Autodesk Fusion 360 part; units mm, degrees
(part 2 of 2)
  line L893 (352.3496, 85.2824) -> (352.3435, 85.227)
  line L894 (352.3793, 85.4468) -> (352.3675, 85.3923)
  line L895 (352.3576, 85.3375) -> (352.3496, 85.2824)
  line L896 (352.7563, 83.9952) -> (352.7945, 83.9547)
  line L897 (352.4662, 85.7111) -> (352.4452, 85.6595)
  line L898 (353.1622, 86.4835) -> (353.114, 86.4555)
  line L899 (352.618, 84.1698) -> (352.6503, 84.1244)
  line L900 (352.3393, 85.1714) -> (352.337, 85.1158)
  line L901 (352.7945, 83.9547) -> (352.8342, 83.9156)
  line L902 (352.5309, 84.3124) -> (352.5583, 84.2639)
  line L903 (352.3367, 85.06) -> (352.3383, 85.0043)
  line L904 (352.6286, 86.0027) -> (352.5974, 85.9565)
  line L905 (353.0206, 86.3947) -> (352.9756, 86.3619)
  line L906 (352.4386, 84.5151) -> (352.459, 84.4632)
  line L907 (354.279, 83.5057) -> (354.3337, 83.5183)
  line L908 (273.0588, 85.3008) -> (273.0502, 85.3558)
  line L909 (355.0618, 83.9218) -> (355.1015, 83.9615)
  line L910 (354.8899, 83.7776) -> (354.9347, 83.8114)
  line L911 (354.6496, 83.6333) -> (354.6996, 83.6587)
  line L912 (355.544, 84.9105) -> (355.5489, 84.9664)
  line L913 (353.7225, 83.4859) -> (353.7778, 83.4792)
  line L914 (354.3879, 83.5328) -> (354.4416, 83.5492)
  line L915 (354.7487, 83.686) -> (354.7969, 83.7149)
  line L916 (355.2119, 84.0886) -> (355.2457, 84.1334)
  line L917 (355.5518, 85.0225) -> (355.5528, 85.0786)
  line L918 (353.3986, 83.5661) -> (353.4513, 83.5481)
  line L919 (355.505, 84.6896) -> (355.5176, 84.7443)
  line L920 (273.0656, 85.2455) -> (273.0588, 85.3008)
  line L921 (355.5371, 84.8548) -> (355.544, 84.9105)
  line L922 (353.5046, 83.5319) -> (353.5585, 83.5176)
  line L923 (273.0704, 85.19) -> (273.0656, 85.2455)
  line L924 (355.5176, 84.7443) -> (355.5284, 84.7994)
  line L925 (353.9447, 83.4705) -> (354.0008, 83.4715)
  line L926 (355.1397, 84.0026) -> (355.1766, 84.045)
  line L927 (353.4513, 83.5481) -> (353.5046, 83.5319)
  line L928 (354.1685, 83.4862) -> (354.2239, 83.4949)
  line L929 (355.39, 84.3737) -> (355.4138, 84.4245)
  line L930 (355.2457, 84.1334) -> (355.2779, 84.1794)
  line L931 (355.5284, 84.7994) -> (355.5371, 84.8548)
  line L932 (354.3337, 83.5183) -> (354.3879, 83.5328)
  line L933 (355.5489, 84.9664) -> (355.5518, 85.0225)
  line L934 (355.2779, 84.1794) -> (355.3084, 84.2265)
  line L935 (355.4138, 84.4245) -> (355.4357, 84.4762)
  line L936 (354.9784, 83.8467) -> (355.0207, 83.8836)
  line L937 (354.1128, 83.4793) -> (354.1685, 83.4862)
  line L938 (354.2239, 83.4949) -> (354.279, 83.5057)
  line L939 (354.6996, 83.6587) -> (354.7487, 83.686)
  line L940 (353.7778, 83.4792) -> (353.8333, 83.4744)
  line L941 (355.4357, 84.4762) -> (355.4558, 84.5286)
  line L942 (353.5585, 83.5176) -> (353.6128, 83.5051)
  line L943 (354.4416, 83.5492) -> (354.4947, 83.5675)
  line L944 (354.9347, 83.8114) -> (354.9784, 83.8467)
  line L945 (354.4947, 83.5675) -> (354.5471, 83.5876)
  line L946 (353.3465, 83.5859) -> (353.3986, 83.5661)
  line L947 (354.5988, 83.6095) -> (354.6496, 83.6333)
  line L948 (355.3084, 84.2265) -> (355.3373, 84.2746)
  line L949 (353.6675, 83.4946) -> (353.7225, 83.4859)
  line L950 (355.4558, 84.5286) -> (355.4741, 84.5817)
  line L951 (354.0008, 83.4715) -> (354.0569, 83.4744)
  line L952 (354.0569, 83.4744) -> (354.1128, 83.4793)
  line L953 (353.6128, 83.5051) -> (353.6675, 83.4946)
  line L954 (353.8333, 83.4744) -> (353.889, 83.4715)
  line L955 (270.6355, 86.4555) -> (270.5883, 86.4259)
  line L956 (271.9772, 86.6034) -> (271.9241, 86.6201)
  line L957 (273.0502, 85.3558) -> (273.0396, 85.4105)
  line L958 (271.2624, 86.6738) -> (271.2073, 86.6657)
  line L959 (272.2809, 86.465) -> (272.2324, 86.4924)
  line L960 (270.3691, 86.2544) -> (270.3291, 86.2157)
  line L961 (273.0743, 85.0786) -> (273.0733, 85.1343)
  line L962 (272.7033, 86.1059) -> (272.667, 86.1482)
  line L963 (354.8439, 83.7454) -> (354.8899, 83.7776)
  line L964 (355.0207, 83.8836) -> (355.0618, 83.9218)
  line L965 (273.0129, 85.5187) -> (272.9967, 85.572)
  line L966 (355.4905, 84.6354) -> (355.505, 84.6896)
  line L967 (354.5471, 83.5876) -> (354.5988, 83.6095)
  line L968 (355.3646, 84.3237) -> (355.39, 84.3737)
  line L969 (272.9139, 85.7787) -> (272.8887, 85.8285)
  line L970 (272.9589, 85.6768) -> (272.9372, 85.7282)
  line L971 (272.0816, 86.5643) -> (272.0297, 86.5847)
  line L972 (271.8704, 86.6351) -> (271.8162, 86.6481)
  line L973 (355.3373, 84.2746) -> (355.3646, 84.3237)
  line L974 (270.4971, 86.3619) -> (270.4532, 86.3276)
  line L975 (353.889, 83.4715) -> (353.9447, 83.4705)
  line L976 (270.4105, 86.2917) -> (270.3691, 86.2544)
  line L977 (353.2951, 83.6075) -> (353.3465, 83.5859)
  line L978 (272.183, 86.5181) -> (272.1327, 86.5421)
  line L979 (270.9376, 86.5973) -> (270.8853, 86.5781)
  line L980 (355.1766, 84.045) -> (355.2119, 84.0886)
  line L981 (270.4532, 86.3276) -> (270.4105, 86.2917)
  line L982 (271.3178, 86.6799) -> (271.2624, 86.6738)
  line L983 (272.4646, 86.3392) -> (272.4204, 86.373)
  line L984 (355.4741, 84.5817) -> (355.4905, 84.6354)
  line L985 (270.5883, 86.4259) -> (270.5421, 86.3947)
  line L986 (272.9967, 85.572) -> (272.9787, 85.6247)
  line L987 (273.0733, 85.1343) -> (273.0704, 85.19)
  line L988 (272.5901, 86.2288) -> (272.5495, 86.267)
  line L989 (272.6292, 86.1891) -> (272.5901, 86.2288)
  line L990 (272.5077, 86.3038) -> (272.4646, 86.3392)
  line L991 (272.2324, 86.4924) -> (272.183, 86.5181)
  line L992 (273.0396, 85.4105) -> (273.0272, 85.4648)
  line L993 (271.9241, 86.6201) -> (271.8704, 86.6351)
  line L994 (271.6515, 86.676) -> (271.596, 86.6815)
  line L995 (271.098, 86.644) -> (271.044, 86.6303)
  line L996 (271.044, 86.6303) -> (270.9905, 86.6147)
  line L997 (270.7828, 86.5343) -> (270.7328, 86.5098)
  line L998 (271.3734, 86.684) -> (271.3178, 86.6799)
  line L999 (272.9787, 85.6247) -> (272.9589, 85.6768)
  line L1000 (270.3291, 86.2157) -> (270.2904, 86.1756)
  line L1001 (272.667, 86.1482) -> (272.6292, 86.1891)
  line L1002 (271.429, 86.6863) -> (271.3734, 86.684)
  line L1003 (272.7715, 86.0178) -> (272.7382, 86.0625)
  line L1004 (270.241, 84.0371) -> (270.2778, 83.9952)
  line L1005 (270.4388, 83.8415) -> (270.4823, 83.8066)
  line L1006 (272.8619, 85.8773) -> (272.8334, 85.9252)
  line L1007 (272.8887, 85.8285) -> (272.8619, 85.8773)
  line L1008 (270.9905, 86.6147) -> (270.9376, 86.5973)
  line L1009 (272.8033, 85.972) -> (272.7715, 86.0178)
  line L1010 (272.7382, 86.0625) -> (272.7033, 86.1059)
  line L1011 (273.0272, 85.4648) -> (273.0129, 85.5187)
  line L1012 (270.6837, 86.4835) -> (270.6355, 86.4555)
  line L1013 (272.3285, 86.436) -> (272.2809, 86.465)
  line L1014 (272.1327, 86.5421) -> (272.0816, 86.5643)
  line L1015 (271.7067, 86.6686) -> (271.6515, 86.676)
  line L1016 (271.2073, 86.6657) -> (271.1524, 86.6558)
  line L1017 (270.7328, 86.5098) -> (270.6837, 86.4835)
  line L1018 (270.5421, 86.3947) -> (270.4971, 86.3619)
  line L1019 (271.7617, 86.6593) -> (271.7067, 86.6686)
  line L1020 (270.8337, 86.5571) -> (270.7828, 86.5343)
  line L1021 (272.5495, 86.267) -> (272.5077, 86.3038)
  line L1022 (271.8162, 86.6481) -> (271.7617, 86.6593)
  line L1023 (271.4847, 86.6866) -> (271.429, 86.6863)
  line L1024 (270.8853, 86.5781) -> (270.8337, 86.5571)
  line L1025 (271.5404, 86.685) -> (271.4847, 86.6866)
  line L1026 (272.375, 86.4053) -> (272.3285, 86.436)
  line L1027 (272.0297, 86.5847) -> (271.9772, 86.6034)
  line L1028 (271.596, 86.6815) -> (271.5404, 86.685)
  line L1029 (272.4204, 86.373) -> (272.375, 86.4053)
  line L1030 (272.8334, 85.9252) -> (272.8033, 85.972)
  line L1031 (271.1524, 86.6558) -> (271.098, 86.644)
  line L1032 (272.9372, 85.7282) -> (272.9139, 85.7787)
  line L1033 (324.4951, 91.4174) -> (324.4508, 91.4512)
  line L1034 (323.7372, 91.7468) -> (323.6819, 91.7542)
  line L1035 (323.5152, 91.7648) -> (323.4595, 91.7645)
  line L1036 (273.8925, 132.1833) -> (273.9308, 132.2244)
  line L1037 (325.096, 90.3237) -> (325.0893, 90.379)
  line L1038 (324.5382, 91.382) -> (324.4951, 91.4174)
  line L1039 (323.6265, 91.7597) -> (323.5709, 91.7632)
  line L1040 (323.3482, 91.7581) -> (323.2929, 91.752)
  line L1041 (323.9545, 91.6983) -> (323.9009, 91.7133)
  line L1042 (274.335, 133.1323) -> (274.3399, 133.1882)
  line L1043 (323.8467, 91.7264) -> (323.7921, 91.7375)
  line L1044 (324.6205, 91.307) -> (324.58, 91.3452)
  line L1045 (274.2815, 132.8572) -> (274.2961, 132.9114)
  line L1046 (273.8528, 132.1436) -> (273.8925, 132.1833)
  line L1047 (274.1556, 132.5455) -> (274.1811, 132.5955)
  line L1048 (323.5709, 91.7632) -> (323.5152, 91.7648)
  line L1049 (324.0602, 91.6629) -> (324.0077, 91.6816)
  line L1050 (324.2134, 91.5963) -> (324.1631, 91.6203)
  line L1051 (274.3087, 132.9661) -> (274.3194, 133.0212)
  line L1052 (274.1811, 132.5955) -> (274.2048, 132.6463)
  line L1053 (274.2267, 132.698) -> (274.2468, 132.7504)
  line L1054 (274.2048, 132.6463) -> (274.2267, 132.698)
  line L1055 (274.0029, 132.3104) -> (274.0367, 132.3552)
  line L1056 (274.3399, 133.1882) -> (274.3428, 133.2443)
  line L1057 (274.2651, 132.8035) -> (274.2815, 132.8572)
  line L1058 (273.9676, 132.2667) -> (274.0029, 132.3104)
  line L1059 (274.0367, 132.3552) -> (274.0689, 132.4012)
  line L1060 (324.4508, 91.4512) -> (324.4054, 91.4835)
  line L1061 (274.2468, 132.7504) -> (274.2651, 132.8035)
  line L1062 (325.0893, 90.379) -> (325.0806, 90.434)
  line L1063 (324.112, 91.6425) -> (324.0602, 91.6629)
  line L1064 (273.9308, 132.2244) -> (273.9676, 132.2667)
  line L1065 (274.2961, 132.9114) -> (274.3087, 132.9661)
  line L1066 (325.0272, 90.6502) -> (325.0091, 90.7029)
  line L1067 (273.8117, 132.1054) -> (273.8528, 132.1436)
  line L1068 (274.3194, 133.0212) -> (274.3282, 133.0766)
  line L1069 (274.3428, 133.2443) -> (274.3438, 133.3004)
  line L1070 (323.6819, 91.7542) -> (323.6265, 91.7597)
  line L1071 (324.9443, 90.8569) -> (324.9192, 90.9067)
  line L1072 (274.0689, 132.4012) -> (274.0995, 132.4482)
  line L1073 (274.1284, 132.4964) -> (274.1556, 132.5455)
  line L1074 (274.3282, 133.0766) -> (274.335, 133.1323)
  line L1075 (274.0995, 132.4482) -> (274.1284, 132.4964)
  line L1076 (324.3114, 91.5432) -> (324.2628, 91.5706)
  line L1077 (325.0091, 90.7029) -> (324.9893, 90.755)
  line L1078 (324.9677, 90.8064) -> (324.9443, 90.8569)
  line L1079 (324.2628, 91.5706) -> (324.2134, 91.5963)
  line L1080 (324.0077, 91.6816) -> (323.9545, 91.6983)
  line L1081 (322.8641, 91.6353) -> (322.8133, 91.6125)
  line L1082 (324.8337, 91.0502) -> (324.8019, 91.096)
  line L1083 (324.8019, 91.096) -> (324.7686, 91.1407)
  line L1084 (323.4038, 91.7622) -> (323.3482, 91.7581)
  line L1085 (323.9009, 91.7133) -> (323.8467, 91.7264)
  line L1086 (324.6974, 91.2264) -> (324.6597, 91.2674)
  line L1087 (325.0806, 90.434) -> (325.0701, 90.4887)
  line L1088 (325.0701, 90.4887) -> (325.0576, 90.5431)
  line L1089 (324.6597, 91.2674) -> (324.6205, 91.307)
  line L1090 (324.8924, 90.9555) -> (324.8638, 91.0034)
  line L1091 (323.4595, 91.7645) -> (323.4038, 91.7622)
  line L1092 (325.1009, 90.2682) -> (325.096, 90.3237)
  line L1093 (325.0433, 90.5969) -> (325.0272, 90.6502)
  line L1094 (324.9192, 90.9067) -> (324.8924, 90.9555)
  line L1095 (324.58, 91.3452) -> (324.5382, 91.382)
  line L1096 (324.8638, 91.0034) -> (324.8337, 91.0502)
  line L1097 (325.1037, 90.2125) -> (325.1009, 90.2682)
  line L1098 (324.1631, 91.6203) -> (324.112, 91.6425)
  line L1099 (322.0828, 89.3906) -> (322.1102, 89.3421)
  line L1100 (321.9066, 89.9163) -> (321.9159, 89.8613)
  line L1101 (322.0409, 90.8402) -> (322.0181, 90.7893)
  line L1102 (324.3589, 91.5142) -> (324.3114, 91.5432)
  line L1103 (324.4054, 91.4835) -> (324.3589, 91.5142)
  line L1104 (322.3208, 91.2538) -> (322.2835, 91.2125)
  line L1105 (323.7921, 91.7375) -> (323.7372, 91.7468)
  line L1106 (324.7686, 91.1407) -> (324.7338, 91.1842)
  line L1107 (325.0576, 90.5431) -> (325.0433, 90.5969)
  line L1108 (325.1047, 90.1568) -> (325.1037, 90.2125)
  line L1109 (324.9893, 90.755) -> (324.9677, 90.8064)
  line L1110 (322.0571, 89.44) -> (322.0828, 89.3906)
  line L1111 (322.1493, 91.0347) -> (322.1197, 90.9875)
  line L1112 (324.7338, 91.1842) -> (324.6974, 91.2264)
sketch "Sketch2" plane through (0, 0, 0) normal (1, 0, 0) x (0, 1, 0)
  line L0 (54.1902, 0) -> (10.8152, -20.7484)
  line L1 (0, 0) -> (10.8152, -20.7484)
  point P0 (0.8902, 0)
  point P1 (54.1902, 0)
  constraint coincident P1 L0.start
  constraint coincident L1.start origin
sketch "Sketch3" plane through (0, 0, 0) normal (1, 0, 0) x (0, 1, 0)
  line L0 (54.1902, 0) -> (10.8152, -20.7484)
  line L1 (10.8152, -20.7484) -> (12.6194, -19.8853)
  line L2 (12.6194, -19.8853) -> (11.7563, -18.0811)
  line L3 (0, 0) -> (10.8152, -20.7484)
  line L4 (11.7563, -18.0811) -> (9.8902, -18.9738)
  line L5 (1.6308, 0) -> (1.398, 0)
  line L6 (0, 0) -> (2, 0)
  line L7 (11.7563, -18.0811) -> (2, 0)
  line L8 (51.1011, 0) -> (51.1542, 0)
  line L9 (54.1902, 0) -> (52.1902, 0)
  line L10 (1.8847, 0) -> (53.1746, 0)
  line L11 (11.7563, -18.0811) -> (48.152, 0)
  line L12 (48.152, 0) -> (48.152, -2.8884)
  line L13 (48.152, -2.8884) -> (1.5056, -2.8884)
  point P0 (10.8152, -20.7484)
  dimension "d2" = 2
  dimension "d3" = 2
  dimension "d4" = 2
  dimension "d5" = 2
  constraint coincident P0 L0.end
  constraint coincident L0 L1.end
  constraint perpendicular L0 L2
  constraint coincident L3 L4.end
  constraint perpendicular L2 L4
  constraint coincident L3.start L6.start
  constraint parallel L5 L6
  constraint coincident L0.start L9.start
  constraint parallel L8 L9
  constraint coincident L10 L11.end
  constraint coincident L0 L12.end
  constraint perpendicular L10 L12
  constraint coincident L3 L13.end
  constraint perpendicular L12 L13
  measures "d2" distance of P0 L1.end
  measures "d3" distance of L1.end L2.end
  measures "d4" distance of L3.start L6.end
  measures "d5" distance of L0.start L9.end
extrude "Extrude1" add sketch "Sketch3" along normal blind 99 contours L0 L8 L9 L10 L12 | L11 L12 L13 | L0 L2 L11 L13 | L0 L1 L2 L3 L4 | L7 L10 L11 L13 | L3 L4 L7 L13 | L3 L5 L6 L7 L10 L13
extrude "Extrude2" cut 1 faces at (0, 30.83, -0.9628) along direction (1, 0, 0) blind 61
sketch "Sketch4" plane through (0, 0, 0) normal (0, 0, 1) x (-1, 0, 0)
  line L0 (-61, -54.1902) -> (-61, 0)
  line L1 (-61, 0) -> (-99, 0)
  line L2 (-99, 0) -> (-99, -54.1902)
  line L3 (-99, -54.1902) -> (-61, -54.1902)
  line L4 (-61, -0.8841) -> (-99, -0.8876)
  constraint coincident L0 L4.start
  constraint coincident L2 L4.end
extrude "Extrude3" cut sketch "Sketch4" against normal blind 10 contours L0 L1 L2 L4
extrude "Extrude5" cut sketch "dimensioniMega" against normal blind 24 contours L585 L587 L590 L591 L592 L594 L595 L596 L597 L598 L599 L600 L602 L603 L604 L605 L608 L609 L611 L612 L613 L614 L615 L616 L619 L620 L622 L623 L624 L626 L627 L628 L630 L631 L632 L633 L634 L635 L636 L637 L638 L639 L641 L642 L643 L644 L645 L646 L647 L648 L649 L651 L652 L653 L654 L655 L656 L657 L658 L659 L660 L661 L662 L663 L664 L665 L666 L667 L668 L669 L670 L671 L672 L673 L674 L675 L676 L677 L678 L679 L680 L681 L682 L683 L684 L685 L686 L687 L688 L689 L690 L691 L692 L693 L694 L695 L696 L697 L698 L699 L700 L701 L702 L703 L704 L705 L706 L707 L708 L709 L710 L711 L712 L713 L714 L715 L716 L717 L718 L719 L720 L721 L722 L723 L724 L725 L726 L727 L728 L729 L730 L731 L732 L733 L734 L735 L736 L737 L738 L739 L740 L741 L742 L743 L744 L745 L746 L747 L748 L749 L750 L751 L752 L753 L754 L755 L756 L757 L758 L759 L760 L761 L762 L763 L764 L765 L766 L767 L768 L769 L770 L771 L772 L773 L774 L775 L776 L794 L801 L821 L825
extrude "Extrude6" cut sketch "dimensioniMega" against normal blind 17 contours L777 L778 L779 L780 L781 L782 L783 L784 L785 L786 L787 L788 L789 L790 L791 L792 L793 L795 L796 L797 L798 L799 L800 L802 L803 L804 L805 L806 L807 L808 L809 L810 L811 L812 L813 L814 L815 L816 L817 L818 L819 L820 L822 L823 L824 L826 L827 L828 L829 L830 L831 L832 L833 L834 L835 L836 L837 L838 L839 L840 L841 L842 L843 L844 L845 L846 L847 L848 L849 L850 L851 L852 L853 L854 L855 L856 L857 L858 L859 L860 L861 L862 L863 L864 L865 L866 L867 L868 L869 L870 L871 L872 L873 L874 L875 L876 L877 L878 L879 L880 L881 L882 L883 L884 L885 L886 L887 L888 L889 L890 L891 L892 L893 L894 L895 L896 L897 L898 L899 L900 L901 L902 L903 L904 L905 L906 L907 L909 L910 L911 L912 L913 L914 L915 L916 L917 L918 L919 L921 L922 L924 L925 L926 L927 L928 L929 L930 L931 L932 L933 L934 L935 L936 L937 L938 L939 L940 L941 L942 L943 L944 L945 L946 L947 L948 L949 L950 L951 L952 L953 L954 L963 L964 L966 L967 L968 L973 L975 L977 L980 L984
extrude "Extrude7" cut sketch "dimensioniMega" against normal blind 4 contours L294 L295 L296 L297 L298 L299 L300 L301 L302 L303 L304 L305 L306 L307 L308 L309 L310 L311 L312 L313 L314 L315 L316 L317 L318 L319 L320 L321 L322 L323 L324 L325 L326 L327 L328 L329 L330 L331 L332 L333 L334 L335 L336 L337 L338 L339 L340 L341 L342 L343 L344 L345 L346 L347 L348 L349 L350 L351 L352 L353 L354 L355 L356 L357 L358 L359 L360 L361 L362 L363 L364 L365 L366 L367 L368 L369 L370 L371 L372 L373 L374 L375 L376 L377 L378 L379 L380 L381 L382 L383 L384 L385 L386 L387 L388 L389 L390 L391 L392 L393 L394 L395 L396 L397 L398 L399 L400 L401 L402 L403 L404 L405 L406 L407 L408 L409 L410 L411 L424 L426 L446 L455 L461 L463 L467 L1033 L1034 L1035 L1037 L1038 L1039 L1040 L1041 L1043 L1044 L1048 L1049 L1050 L1060 L1062 L1063 L1066 L1070 L1071 L1076 L1077 L1078 L1079 L1080 L1081 L1082 L1083 L1084 L1085 L1086 L1087 L1088 L1089 L1090 L1091 L1092 L1093 L1094 L1095 L1096 L1097 L1098 L1099 L1100 L1101 L1102 L1103 L1104 L1105 L1106 L1107 L1108 L1109 L1110 L1111 L1112 | L412 L413 L414 L415 L416 L417 L418 L419 L420 L421 L422 L423 L425 L427 L428 L429 L430 L431 L432 L433 L434 L435 L436 L437 L438 L439 L440 L441 L442 L443 L444 L445 L447 L448 L449 L450 L451 L452 L453 L454 L456 L457 L458 L459 L460 L462 L464 L465 L466 L468 L469 L470 L471 L472 L473 L474 L475 L476 L477 L478 L479 L480 L481 L482 L483 L484 L485 L486 L487 L488 L489 L490 L491 L492 L493 L494 L495 L496 L497 L498 L499 L500 L501 L502 L503 L504 L505 L506 L507 L508 L509 L510 L511 L512 L513 L514 L515 L516 L517 L518 L519 L520 L521 L522 L523 L524 L525 L526 L527 L528 L529 L530 L531 L532 L533 L534 L535 L536 L537 L538 L539 L540 L541 L542 L543 L544 L545 L546 L547 L548 L549 L550 L551 L552 L553 L554 L555 L556 L557 L558 L559 L560 L561 L562 L563 L564 L565 L566 L567 L568 L569 L570 L571 L572 L573 L574 L575 L576 L577 L578 L579 L580 L581 L582 L583 L584 L586 L588 L589 L593 L601 L606 L607 L610 L617 L618 L621 L625 L629 L640 L650
